Autodesk Fusion 360 part; units mm, degrees
note: some values were not read from the file. Set by a fixed rule: which sketch regions a step uses.
(part 3 of 4)
sketch "スケッチ30" plane through (0, 0, 3) normal (0, 0, 1) x (-1, 0, 0)
  arc A0 (40, -80.2208) -> (44, -84.2208) centre (44, -80.2208) ccw
  line L0 (44, -84.2208) -> (61.0153, -84.2208)
  arc A1 (61.0153, -84.2208) -> (67.021, -79.5248) centre (0, 0) ccw
  arc A2 (67.021, -79.5248) -> (66.4432, -73.002) centre (64.4432, -76.4661) ccw
  line L1 (66.4432, -73.002) -> (56.3605, -67.1808)
  arc A3 (55.6284, -64.4487) -> (56.3605, -67.1808) centre (57.3605, -65.4487) ccw
  line L2 (55.6284, -64.4487) -> (83.6284, -15.9513)
  arc A4 (86.3605, -15.2192) -> (83.6284, -15.9513) centre (85.3605, -16.9513) ccw
  line L3 (86.3605, -15.2192) -> (96.4432, -21.0405)
  arc A5 (96.4432, -21.0405) -> (102.381, -18.2795) centre (98.4432, -17.5764) ccw
  arc A6 (102.381, -18.2795) -> (94.1613, 44.1547) centre (0, 0) ccw
  arc A7 (94.1613, 44.1547) -> (87.7113, 45.2849) centre (90.5398, 42.4565) ccw
  line L4 (87.7113, 45.2849) -> (79.4788, 37.0524)
  arc A8 (76.6504, 37.0524) -> (79.4788, 37.0524) centre (78.0646, 38.4666) ccw
  line L5 (76.6504, 37.0524) -> (37.0524, 76.6504)
  arc A9 (37.0524, 79.4788) -> (37.0524, 76.6504) centre (38.4666, 78.0646) ccw
  line L6 (37.0524, 79.4788) -> (45.2849, 87.7113)
  arc A10 (45.2849, 87.7113) -> (44.1547, 94.1613) centre (42.4565, 90.5398) ccw
  arc A11 (44.1547, 94.1613) -> (-44.1547, 94.1613) centre (0, 0) ccw
  arc A12 (-44.1547, 94.1613) -> (-45.2849, 87.7113) centre (-42.4565, 90.5398) ccw
  line L7 (-45.2849, 87.7113) -> (-37.0524, 79.4788)
  arc A13 (-37.0524, 76.6504) -> (-37.0524, 79.4788) centre (-38.4666, 78.0646) ccw
  line L8 (-37.0524, 76.6504) -> (-76.6504, 37.0524)
  arc A14 (-79.4788, 37.0524) -> (-76.6504, 37.0524) centre (-78.0646, 38.4666) ccw
  line L9 (-79.4788, 37.0524) -> (-87.7113, 45.2849)
  arc A15 (-87.7113, 45.2849) -> (-94.1613, 44.1547) centre (-90.5398, 42.4565) ccw
  arc A16 (-94.1613, 44.1547) -> (-102.381, -18.2795) centre (0, 0) ccw
  arc A17 (-102.381, -18.2795) -> (-96.4432, -21.0405) centre (-98.4432, -17.5764) ccw
  line L10 (-96.4432, -21.0405) -> (-86.3605, -15.2192)
  arc A18 (-83.6284, -15.9513) -> (-86.3605, -15.2192) centre (-85.3605, -16.9513) ccw
  line L11 (-83.6284, -15.9513) -> (-55.6284, -64.4487)
  arc A19 (-56.3605, -67.1808) -> (-55.6284, -64.4487) centre (-57.3605, -65.4487) ccw
  line L12 (-56.3605, -67.1808) -> (-66.4432, -73.002)
  arc A20 (-66.4432, -73.002) -> (-67.021, -79.5248) centre (-64.4432, -76.4661) ccw
  arc A21 (-67.021, -79.5248) -> (-61.3188, -84) centre (0, 0) ccw
  line L13 (-61.3188, -84) -> (-44, -84)
  arc A22 (-44, -84) -> (-40, -80) centre (-44, -80) ccw
  line L14 (-40, -80) -> (-40, -66)
  arc A23 (-38, -64) -> (-40, -66) centre (-38, -66) ccw
  line L15 (-38, -64) -> (38, -64)
  arc A24 (40, -66) -> (38, -64) centre (38, -66) ccw
  line L16 (40, -66) -> (40, -80.2208)
  arc A25 (-4, -46.6154) -> (-5.7447, -44.6318) centre (-6, -46.6154) ccw
  arc A26 (-28.3589, -34.9396) -> (-5.7447, -44.6318) centre (0, 0) ccw
  arc A27 (-28.4908, -31.9509) -> (-28.3589, -34.9396) centre (-27.0985, -33.3867) ccw
  line L17 (-28.4908, -31.9509) -> (-25.5966, -29.1445)
  arc A28 (-22.9631, -29.012) -> (-25.5966, -29.1445) centre (-24.2043, -30.5803) ccw
  arc A29 (-22.9631, -29.012) -> (22.9694, -29.007) centre (0, 0) ccw
  arc A30 (25.6252, -29.1607) -> (22.9694, -29.007) centre (24.211, -30.575) ccw
  line L18 (25.6252, -29.1607) -> (28.4709, -32.0064)
  arc A31 (28.3151, -34.9751) -> (28.4709, -32.0064) centre (27.0567, -33.4206) ccw
  arc A32 (5.7447, -44.6318) -> (28.3151, -34.9751) centre (0, 0) ccw
  arc A33 (5.7447, -44.6318) -> (4, -46.6154) centre (6, -46.6154) ccw
  line L19 (4, -46.6154) -> (4, -48)
  arc A34 (4, -48) -> (6, -50) centre (6, -48) ccw
  line L20 (6, -50) -> (38, -50)
  arc A35 (40, -52) -> (38, -50) centre (38, -52) ccw
  line L21 (40, -52) -> (40, -56)
  arc A36 (38, -58) -> (40, -56) centre (38, -56) ccw
  line L22 (38, -58) -> (-38, -58)
  arc A37 (-40, -56) -> (-38, -58) centre (-38, -56) ccw
  line L23 (-40, -56) -> (-40, -52)
  arc A38 (-38, -50) -> (-40, -52) centre (-38, -52) ccw
  line L24 (-38, -50) -> (-6, -50)
  arc A39 (-6, -50) -> (-4, -48) centre (-6, -48) ccw
  line L25 (-4, -48) -> (-4, -47)
  line L26 (-4, -47) -> (-4, -46.6154)
  line L27 (55.9233, -53.938) -> (50.6914, -63)
  arc A40 (48.9593, -64) -> (50.6914, -63) centre (48.9593, -62) ccw
  line L28 (48.9593, -64) -> (47, -64)
  arc A41 (45, -62) -> (47, -64) centre (47, -62) ccw
  line L29 (45, -62) -> (45, -51.9629)
  arc A42 (46.9625, -49.9632) -> (45, -51.9629) centre (47, -51.9629) ccw
  line L30 (46.9625, -49.9632) -> (52.2919, -49.8634)
  arc A43 (53.3294, -50.131) -> (52.2919, -49.8634) centre (52.3294, -51.863) ccw
  line L31 (53.3294, -50.131) -> (55.1913, -51.2059)
  arc A44 (55.9233, -53.938) -> (55.1913, -51.2059) centre (54.1913, -52.938) ccw
  line L32 (-52.5666, -50) -> (-47, -50)
  arc A45 (-45, -52) -> (-47, -50) centre (-47, -52) ccw
  line L33 (-45, -52) -> (-45, -62)
  arc A46 (-47, -64) -> (-45, -62) centre (-47, -62) ccw
  line L34 (-47, -64) -> (-48.9593, -64)
  arc A47 (-50.6914, -63) -> (-48.9593, -64) centre (-48.9593, -62) ccw
  line L35 (-50.6914, -63) -> (-55.9233, -53.938)
  arc A48 (-55.1913, -51.2059) -> (-55.9233, -53.938) centre (-54.1913, -52.938) ccw
  line L36 (-55.1913, -51.2059) -> (-53.5666, -50.2679)
  arc A49 (-52.5666, -50) -> (-53.5666, -50.2679) centre (-52.5666, -52) ccw
  arc A50 (76.6504, 29.9813) -> (79.4788, 29.9813) centre (78.0646, 31.3955) ccw
  line L37 (79.4788, 29.9813) -> (88.1522, 38.6547)
  arc A51 (91.4132, 38.0084) -> (88.1522, 38.6547) centre (89.5664, 37.2405) ccw
  arc A52 (98.3614, 11.2268) -> (91.4132, 38.0084) centre (0, 0) ccw
  arc A53 (96.3743, 9) -> (98.3614, 11.2268) centre (96.3743, 11) ccw
  line L38 (96.3743, 9) -> (50.8232, 9)
  arc A54 (48.8685, 10.5769) -> (50.8232, 9) centre (50.8232, 11) ccw
  arc A55 (48.8685, 10.5769) -> (45.7253, 20.2286) centre (0, 0) ccw
  arc A56 (46.1401, 22.452) -> (45.7253, 20.2286) centre (47.5543, 21.0378) ccw
  line L39 (46.1401, 22.452) -> (63.7457, 40.0576)
  arc A57 (66.5741, 40.0576) -> (63.7457, 40.0576) centre (65.1599, 38.6434) ccw
  line L40 (66.5741, 40.0576) -> (76.6504, 29.9813)
  arc A58 (98.1356, -13.0538) -> (98.3593, -11.2453) centre (0, 0) ccw
  arc A59 (95.1531, -14.5221) -> (98.1356, -13.0538) centre (96.1531, -12.7901) ccw
  line L41 (95.1531, -14.5221) -> (92.084, -12.7502)
  arc A60 (93.084, -9.0182) -> (92.084, -12.7502) centre (93.084, -11.0182) ccw
  line L42 (93.084, -9.0182) -> (96.3722, -9.0182)
  arc A61 (98.3593, -11.2453) -> (96.3722, -9.0182) centre (96.3722, -11.0182) ccw
  line L43 (-96.3722, -9.0182) -> (-93.084, -9.0182)
  arc A62 (-92.084, -12.7502) -> (-93.084, -9.0182) centre (-93.084, -11.0182) ccw
  line L44 (-92.084, -12.7502) -> (-95.1531, -14.5221)
  arc A63 (-98.1356, -13.0538) -> (-95.1531, -14.5221) centre (-96.1531, -12.7901) ccw
  arc A64 (-98.3593, -11.2453) -> (-98.1356, -13.0538) centre (0, 0) ccw
  arc A65 (-96.3722, -9.0182) -> (-98.3593, -11.2453) centre (-96.3722, -11.0182) ccw
  arc A66 (-44.6318, -5.7447) -> (-46.6154, -4) centre (-46.6154, -6) ccw
  line L45 (-46.6154, -4) -> (-96.9794, -4)
  arc A67 (-98.979, -2.0412) -> (-96.9794, -4) centre (-96.9794, -2) ccw
  arc A68 (-98.979, 2.0412) -> (-98.979, -2.0412) centre (0, 0) ccw
  arc A69 (-96.9794, 4) -> (-98.979, 2.0412) centre (-96.9794, 2) ccw
  line L46 (-96.9794, 4) -> (-46.6154, 4)
  arc A70 (-46.6154, 4) -> (-44.6318, 5.7447) centre (-46.6154, 6) ccw
  arc A71 (-34.9648, 28.3278) -> (-44.6318, 5.7447) centre (0, 0) ccw
  arc A72 (-31.975, 28.4611) -> (-34.9648, 28.3278) centre (-33.4108, 27.0688) ccw
  line L47 (-31.975, 28.4611) -> (-29.1682, 25.5666)
  arc A73 (-29.0345, 22.9346) -> (-29.1682, 25.5666) centre (-30.604, 24.1743) ccw
  arc A74 (-29.0345, 22.9346) -> (-29.007, -22.9694) centre (0, 0) ccw
  arc A75 (-29.1607, -25.6252) -> (-29.007, -22.9694) centre (-30.575, -24.211) ccw
  line L48 (-29.1607, -25.6252) -> (-32.0064, -28.4709)
  arc A76 (-34.9751, -28.3151) -> (-32.0064, -28.4709) centre (-33.4206, -27.0567) ccw
  arc A77 (-44.6318, -5.7447) -> (-34.9751, -28.3151) centre (0, 0) ccw
  line L49 (27.8089, 44.4259) -> (43.5931, 60.2101)
  arc A78 (46.4216, 60.2101) -> (43.5931, 60.2101) centre (45.0073, 58.7959) ccw
  line L50 (46.4216, 60.2101) -> (60.2101, 46.4216)
  arc A79 (60.2101, 43.5931) -> (60.2101, 46.4216) centre (58.7959, 45.0073) ccw
  line L51 (60.2101, 43.5931) -> (44.4259, 27.8089)
  arc A80 (41.3574, 28.0992) -> (44.4259, 27.8089) centre (43.0117, 29.2231) ccw
  arc A81 (41.3574, 28.0992) -> (28.0992, 41.3574) centre (0, 0) ccw
  arc A82 (27.8089, 44.4259) -> (28.0992, 41.3574) centre (29.2231, 43.0117) ccw
  line L52 (-38.3596, -35.7147) -> (-57.6913, -46.8758)
  arc A83 (-60.4233, -46.1437) -> (-57.6913, -46.8758) centre (-58.6913, -45.1437) ccw
  line L53 (-60.4233, -46.1437) -> (-70.1733, -29.2563)
  arc A84 (-69.4413, -26.5242) -> (-70.1733, -29.2563) centre (-68.4413, -28.2563) ccw
  line L54 (-69.4413, -26.5242) -> (-50.1096, -15.3631)
  arc A85 (-47.2208, -16.4376) -> (-50.1096, -15.3631) centre (-49.1096, -17.0951) ccw
  arc A86 (-47.2208, -16.4376) -> (-37.8458, -32.6756) centre (0, 0) ccw
  arc A87 (-38.3596, -35.7147) -> (-37.8458, -32.6756) centre (-39.3596, -33.9826) ccw
  arc A88 (-31.3739, -38.9317) -> (-28.1158, -41.3462) centre (0, 0) ccw
  arc A89 (-29.2404, -45) -> (-28.1158, -41.3462) centre (-29.2404, -43) ccw
  line L55 (-29.2404, -45) -> (-36.9782, -45)
  arc A90 (-37.9782, -41.2679) -> (-36.9782, -45) centre (-36.9782, -43) ccw
  line L56 (-37.9782, -41.2679) -> (-33.6289, -38.7569)
  arc A91 (-31.3739, -38.9317) -> (-33.6289, -38.7569) centre (-32.6289, -40.4889) ccw
  line L57 (80.1362, -12) -> (74.6733, -21.462)
  arc A92 (71.9413, -22.1941) -> (74.6733, -21.462) centre (72.9413, -20.462) ccw
  line L58 (71.9413, -22.1941) -> (55.6136, -12.7673)
  arc A93 (56.6098, -9.0353) -> (55.6136, -12.7673) centre (56.6136, -11.0353) ccw
  line L59 (56.6098, -9.0353) -> (75, -9)
  line L60 (75, -9) -> (78.4042, -9)
  arc A94 (80.1362, -12) -> (78.4042, -9) centre (78.4042, -11) ccw
  line L61 (-44.4259, 27.8089) -> (-60.2101, 43.5931)
  arc A95 (-60.2101, 46.4216) -> (-60.2101, 43.5931) centre (-58.7959, 45.0073) ccw
  line L62 (-60.2101, 46.4216) -> (-46.4216, 60.2101)
  arc A96 (-43.5931, 60.2101) -> (-46.4216, 60.2101) centre (-45.0073, 58.7959) ccw
  line L63 (-43.5931, 60.2101) -> (-27.8089, 44.4259)
  arc A97 (-28.0992, 41.3574) -> (-27.8089, 44.4259) centre (-29.2231, 43.0117) ccw
  arc A98 (-28.0992, 41.3574) -> (-41.3574, 28.0992) centre (0, 0) ccw
  arc A99 (-44.4259, 27.8089) -> (-41.3574, 28.0992) centre (-43.0117, 29.2231) ccw
  line L64 (50.1096, -15.3631) -> (69.4413, -26.5242)
  arc A100 (70.1733, -29.2563) -> (69.4413, -26.5242) centre (68.4413, -28.2563) ccw
  line L65 (70.1733, -29.2563) -> (60.4233, -46.1437)
  arc A101 (57.6913, -46.8758) -> (60.4233, -46.1437) centre (58.6913, -45.1437) ccw
  line L66 (57.6913, -46.8758) -> (38.3596, -35.7147)
  arc A102 (37.8458, -32.6756) -> (38.3596, -35.7147) centre (39.3596, -33.9826) ccw
  arc A103 (37.8458, -32.6756) -> (47.2208, -16.4376) centre (0, 0) ccw
  arc A104 (50.1096, -15.3631) -> (47.2208, -16.4376) centre (49.1096, -17.0951) ccw
  line L67 (-78.4041, -8.9935) -> (-56.6098, -9.0353)
  arc A105 (-55.6136, -12.7673) -> (-56.6098, -9.0353) centre (-56.6136, -11.0353) ccw
  line L68 (-55.6136, -12.7673) -> (-71.9413, -22.1941)
  arc A106 (-74.6733, -21.462) -> (-71.9413, -22.1941) centre (-72.9413, -20.462) ccw
  line L69 (-74.6733, -21.462) -> (-80.14, -11.9935)
  arc A107 (-78.4041, -8.9935) -> (-80.14, -11.9935) centre (-78.4079, -10.9935) ccw
  line L70 (33.6289, -38.7569) -> (37.9782, -41.268)
  arc A108 (36.9782, -45) -> (37.9782, -41.268) centre (36.9782, -43) ccw
  line L71 (36.9782, -45) -> (29.2404, -45)
  arc A109 (28.1158, -41.3462) -> (29.2404, -45) centre (29.2404, -43) ccw
  arc A110 (28.1158, -41.3462) -> (31.3739, -38.9317) centre (0, 0) ccw
  arc A111 (33.6289, -38.7569) -> (31.3739, -38.9317) centre (32.6289, -40.4889) ccw
  circle A112 centre (0, 0) radius 32
  circle A113 centre (-51.2451, -46.0409) radius 1.5
  circle A114 centre (51.2451, -46.0409) radius 1.5
  circle A115 centre (-65.4951, -21.3591) radius 1.5
  circle A116 centre (-57.7353, 37.5827) radius 1.5
  circle A117 centre (-37.5827, 57.7353) radius 1.5
  circle A118 centre (37.5827, 57.7353) radius 1.5
  circle A119 centre (57.7353, 37.5827) radius 1.5
  circle A120 centre (65.4951, -21.3591) radius 1.5
  arc A121 (46.6154, -4) -> (44.6318, -5.7447) centre (46.6154, -6) ccw
  arc A122 (34.9751, -28.3151) -> (44.6318, -5.7447) centre (0, 0) ccw
  arc A123 (32.0064, -28.4709) -> (34.9751, -28.3151) centre (33.4206, -27.0567) ccw
  line L72 (32.0064, -28.4709) -> (29.1607, -25.6252)
  arc A124 (29.007, -22.9694) -> (29.1607, -25.6252) centre (30.575, -24.211) ccw
  arc A125 (29.007, -22.9694) -> (29.007, 22.9694) centre (0, 0) ccw
  arc A126 (29.1607, 25.6252) -> (29.007, 22.9694) centre (30.575, 24.211) ccw
  line L73 (29.1607, 25.6252) -> (32.0064, 28.4709)
  arc A127 (34.9751, 28.3151) -> (32.0064, 28.4709) centre (33.4206, 27.0567) ccw
  arc A128 (44.6318, 5.7447) -> (34.9751, 28.3151) centre (0, 0) ccw
  arc A129 (44.6318, 5.7447) -> (46.6154, 4) centre (46.6154, 6) ccw
  line L74 (46.6154, 4) -> (96.9794, 4)
  arc A130 (98.979, 2.0412) -> (96.9794, 4) centre (96.9794, 2) ccw
  arc A131 (98.979, -2.0412) -> (98.979, 2.0412) centre (0, 0) ccw
  arc A132 (96.9794, -4) -> (98.979, -2.0412) centre (96.9794, -2) ccw
  line L75 (96.9794, -4) -> (46.6154, -4)
  arc A133 (-5.7447, 44.6318) -> (-4, 46.6154) centre (-6, 46.6154) ccw
  line L76 (-4, 46.6154) -> (-4, 96.9794)
  arc A134 (-2.0412, 98.979) -> (-4, 96.9794) centre (-2, 96.9794) ccw
  arc A135 (2.0412, 98.979) -> (-2.0412, 98.979) centre (0, 0) ccw
  arc A136 (4, 96.9794) -> (2.0412, 98.979) centre (2, 96.9794) ccw
  line L77 (4, 96.9794) -> (4, 46.6154)
  arc A137 (4, 46.6154) -> (5.7447, 44.6318) centre (6, 46.6154) ccw
  arc A138 (28.3151, 34.9751) -> (5.7447, 44.6318) centre (0, 0) ccw
  arc A139 (28.4709, 32.0064) -> (28.3151, 34.9751) centre (27.0567, 33.4206) ccw
  line L78 (28.4709, 32.0064) -> (25.6252, 29.1607)
  arc A140 (22.9694, 29.007) -> (25.6252, 29.1607) centre (24.211, 30.575) ccw
  arc A141 (22.9694, 29.007) -> (-22.9694, 29.007) centre (0, 0) ccw
  arc A142 (-25.6252, 29.1607) -> (-22.9694, 29.007) centre (-24.211, 30.575) ccw
  line L79 (-25.6252, 29.1607) -> (-28.4709, 32.0064)
  arc A143 (-28.3151, 34.9751) -> (-28.4709, 32.0064) centre (-27.0567, 33.4206) ccw
  arc A144 (-5.7447, 44.6318) -> (-28.3151, 34.9751) centre (0, 0) ccw
  arc A145 (31.3955, 80.893) -> (31.3955, 75.2362) centre (34.224, 78.0646) ccw
  line L80 (31.3955, 75.2362) -> (40.0576, 66.5741)
  arc A146 (40.0576, 63.7457) -> (40.0576, 66.5741) centre (38.6434, 65.1599) ccw
  line L81 (40.0576, 63.7457) -> (22.452, 46.1401)
  arc A147 (20.2286, 45.7253) -> (22.452, 46.1401) centre (21.0378, 47.5543) ccw
  arc A148 (20.2286, 45.7253) -> (10.5769, 48.8685) centre (0, 0) ccw
  arc A149 (9, 50.8232) -> (10.5769, 48.8685) centre (11, 50.8232) ccw
  line L82 (9, 50.8232) -> (9, 96.3743)
  arc A150 (11.2268, 98.3614) -> (9, 96.3743) centre (11, 96.3743) ccw
  arc A151 (38.0084, 91.4132) -> (11.2268, 98.3614) centre (0, 0) ccw
  arc A152 (38.6547, 88.1522) -> (38.0084, 91.4132) centre (37.2405, 89.5664) ccw
  line L83 (38.6547, 88.1522) -> (31.3955, 80.893)
  arc A153 (-31.3955, 75.2362) -> (-31.3955, 80.893) centre (-34.224, 78.0646) ccw
  line L84 (-31.3955, 80.893) -> (-38.6547, 88.1522)
  arc A154 (-38.0084, 91.4132) -> (-38.6547, 88.1522) centre (-37.2405, 89.5664) ccw
  arc A155 (-11.2268, 98.3614) -> (-38.0084, 91.4132) centre (0, 0) ccw
  arc A156 (-9, 96.3743) -> (-11.2268, 98.3614) centre (-11, 96.3743) ccw
  line L85 (-9, 96.3743) -> (-9, 50.8232)
  arc A157 (-10.5769, 48.8685) -> (-9, 50.8232) centre (-11, 50.8232) ccw
  arc A158 (-10.5769, 48.8685) -> (-20.2286, 45.7253) centre (0, 0) ccw
  arc A159 (-22.452, 46.1401) -> (-20.2286, 45.7253) centre (-21.0378, 47.5543) ccw
  line L86 (-22.452, 46.1401) -> (-40.0576, 63.7457)
  arc A160 (-40.0576, 66.5741) -> (-40.0576, 63.7457) centre (-38.6434, 65.1599) ccw
  line L87 (-40.0576, 66.5741) -> (-31.3955, 75.2362)
  arc A161 (-80.893, 31.3955) -> (-75.2362, 31.3955) centre (-78.0646, 34.224) ccw
  line L88 (-75.2362, 31.3955) -> (-66.5741, 40.0576)
  arc A162 (-63.7457, 40.0576) -> (-66.5741, 40.0576) centre (-65.1599, 38.6434) ccw
  line L89 (-63.7457, 40.0576) -> (-46.1401, 22.452)
  arc A163 (-45.7253, 20.2286) -> (-46.1401, 22.452) centre (-47.5543, 21.0378) ccw
  arc A164 (-45.7253, 20.2286) -> (-48.8685, 10.5769) centre (0, 0) ccw
  arc A165 (-50.8232, 9) -> (-48.8685, 10.5769) centre (-50.8232, 11) ccw
  line L90 (-50.8232, 9) -> (-96.3743, 9)
  arc A166 (-98.3614, 11.2268) -> (-96.3743, 9) centre (-96.3743, 11) ccw
  arc A167 (-91.4132, 38.0084) -> (-98.3614, 11.2268) centre (0, 0) ccw
  arc A168 (-88.1522, 38.6547) -> (-91.4132, 38.0084) centre (-89.5664, 37.2405) ccw
  line L91 (-88.1522, 38.6547) -> (-80.893, 31.3955)
  line L92 (0, -64) -> (0, -84)
  line L93 (0, -84) -> (68, -84)
  line L94 (61.3188, -84) -> (60.734, -84.4269)
  line L95 (61.0153, -84.2208) -> (39.7351, -84.2208)
  line L96 (39.7351, -84.2208) -> (39.5, -84)
  constraint midpoint L15 L92.start
  constraint perpendicular L15 L92
  constraint perpendicular L92 L93
  constraint coincident A1 L94.start
  constraint coincident L93 L94.start
  constraint tangent A1 L94
  constraint coincident L0.end A1.start
  constraint parallel L0 L95
  constraint coincident L93 L96.end
delete_face "面を削除4" 1 faces at (-40.4447, 82.0537, 2.5) on bodies 1
extrude "押し出し29" cut sketch "スケッチ30" against normal blind 6 contours A0 L0 A1 L93 L94 L95 | A0 L93 L95 L96 bodies 1
fillet "フィレット31" radius 4 1 edges at (-40, 84, 2.25) on bodies 1
fillet "フィレット32" radius 19.01 1 edges at (61.3188, 84, 2.25) on bodies 1
fillet "フィレット33" radius 19.01 1 edges at (-61.3188, 84, 2.25) on bodies 1
sketch "スケッチ31" plane through (0, 0, 3) normal (0, 0, 1) x (-1, 0, 0)
  arc A0 (54.7686, -84) -> (67.0189, -79.5265) centre (54.7686, -64.99) ccw
  arc A1 (67.0189, -79.5265) -> (67.021, -79.5248) centre (0, 0) ccw
  arc A2 (67.021, -79.5248) -> (66.4432, -73.002) centre (64.4432, -76.4661) ccw
  line L0 (66.4432, -73.002) -> (56.3605, -67.1808)
  arc A3 (55.6284, -64.4487) -> (56.3605, -67.1808) centre (57.3605, -65.4487) ccw
  line L1 (55.6284, -64.4487) -> (83.6284, -15.9513)
  arc A4 (86.3605, -15.2192) -> (83.6284, -15.9513) centre (85.3605, -16.9513) ccw
  line L2 (86.3605, -15.2192) -> (96.4432, -21.0405)
  arc A5 (96.4432, -21.0405) -> (102.381, -18.2795) centre (98.4432, -17.5764) ccw
  arc A6 (102.381, -18.2795) -> (94.1613, 44.1547) centre (0, 0) ccw
  arc A7 (94.1613, 44.1547) -> (87.7113, 45.2849) centre (90.5398, 42.4565) ccw
  line L3 (87.7113, 45.2849) -> (79.4788, 37.0524)
  arc A8 (76.6504, 37.0524) -> (79.4788, 37.0524) centre (78.0646, 38.4666) ccw
  line L4 (76.6504, 37.0524) -> (37.0524, 76.6504)
  arc A9 (37.0524, 79.4788) -> (37.0524, 76.6504) centre (38.4666, 78.0646) ccw
  line L5 (37.0524, 79.4788) -> (45.2849, 87.7113)
  arc A10 (45.2849, 87.7113) -> (44.1547, 94.1613) centre (42.4565, 90.5398) ccw
  arc A11 (44.1547, 94.1613) -> (-44.1547, 94.1613) centre (0, 0) ccw
  arc A12 (-44.1547, 94.1613) -> (-45.2849, 87.7113) centre (-42.4565, 90.5398) ccw
  line L6 (-45.2849, 87.7113) -> (-37.0524, 79.4788)
  arc A13 (-37.0524, 76.6504) -> (-37.0524, 79.4788) centre (-38.4666, 78.0646) ccw
  line L7 (-37.0524, 76.6504) -> (-76.6504, 37.0524)
  arc A14 (-79.4788, 37.0524) -> (-76.6504, 37.0524) centre (-78.0646, 38.4666) ccw
  line L8 (-79.4788, 37.0524) -> (-87.7113, 45.2849)
  arc A15 (-87.7113, 45.2849) -> (-94.1613, 44.1547) centre (-90.5398, 42.4565) ccw
  arc A16 (-94.1613, 44.1547) -> (-102.381, -18.2795) centre (0, 0) ccw
  arc A17 (-102.381, -18.2795) -> (-96.4432, -21.0405) centre (-98.4432, -17.5764) ccw
  line L9 (-96.4432, -21.0405) -> (-86.3605, -15.2192)
  arc A18 (-83.6284, -15.9513) -> (-86.3605, -15.2192) centre (-85.3605, -16.9513) ccw
  line L10 (-83.6284, -15.9513) -> (-55.6284, -64.4487)
  arc A19 (-56.3605, -67.1808) -> (-55.6284, -64.4487) centre (-57.3605, -65.4487) ccw
  line L11 (-56.3605, -67.1808) -> (-66.4432, -73.002)
  arc A20 (-66.4432, -73.002) -> (-67.021, -79.5248) centre (-64.4432, -76.4661) ccw
  arc A21 (-67.021, -79.5248) -> (-67.0189, -79.5265) centre (0.0001, 0.0001) ccw
  arc A22 (-67.0189, -79.5265) -> (-54.7686, -84) centre (-54.7686, -64.99) ccw
  line L12 (-54.7686, -84) -> (-44, -84)
  arc A23 (-44, -84) -> (-40, -80) centre (-44, -80) ccw
  line L13 (-40, -80) -> (-40, -66)
  arc A24 (-38, -64) -> (-40, -66) centre (-38, -66) ccw
  line L14 (-38, -64) -> (38, -64)
  arc A25 (40, -66) -> (38, -64) centre (38, -66) ccw
  line L15 (40, -66) -> (40, -80)
  arc A26 (40, -80) -> (44, -84) centre (44, -80) ccw
  line L16 (44, -84) -> (54.7686, -84)
  arc A27 (-4, -46.6154) -> (-5.7447, -44.6318) centre (-6, -46.6154) ccw
  arc A28 (-28.3589, -34.9396) -> (-5.7447, -44.6318) centre (0, 0) ccw
  arc A29 (-28.4908, -31.9509) -> (-28.3589, -34.9396) centre (-27.0985, -33.3867) ccw
  line L17 (-28.4908, -31.9509) -> (-25.5966, -29.1445)
  arc A30 (-22.9631, -29.012) -> (-25.5966, -29.1445) centre (-24.2043, -30.5803) ccw
  arc A31 (-22.9631, -29.012) -> (22.9694, -29.007) centre (0, 0) ccw
  arc A32 (25.6252, -29.1607) -> (22.9694, -29.007) centre (24.211, -30.575) ccw
  line L18 (25.6252, -29.1607) -> (28.4709, -32.0064)
  arc A33 (28.3151, -34.9751) -> (28.4709, -32.0064) centre (27.0567, -33.4206) ccw
  arc A34 (5.7447, -44.6318) -> (28.3151, -34.9751) centre (0, 0) ccw
  arc A35 (5.7447, -44.6318) -> (4, -46.6154) centre (6, -46.6154) ccw
  line L19 (4, -46.6154) -> (4, -48)
  arc A36 (4, -48) -> (6, -50) centre (6, -48) ccw
  line L20 (6, -50) -> (38, -50)
  arc A37 (40, -52) -> (38, -50) centre (38, -52) ccw
  line L21 (40, -52) -> (40, -56)
  arc A38 (38, -58) -> (40, -56) centre (38, -56) ccw
  line L22 (38, -58) -> (-38, -58)
  arc A39 (-40, -56) -> (-38, -58) centre (-38, -56) ccw
  line L23 (-40, -56) -> (-40, -52)
  arc A40 (-38, -50) -> (-40, -52) centre (-38, -52) ccw
  line L24 (-38, -50) -> (-6, -50)
  arc A41 (-6, -50) -> (-4, -48) centre (-6, -48) ccw
  line L25 (-4, -48) -> (-4, -47)
  line L26 (-4, -47) -> (-4, -46.6154)
  line L27 (55.9233, -53.938) -> (50.6914, -63)
  arc A42 (48.9593, -64) -> (50.6914, -63) centre (48.9593, -62) ccw
  line L28 (48.9593, -64) -> (47, -64)
  arc A43 (45, -62) -> (47, -64) centre (47, -62) ccw
  line L29 (45, -62) -> (45, -51.9629)
  arc A44 (46.9625, -49.9632) -> (45, -51.9629) centre (47, -51.9629) ccw
  line L30 (46.9625, -49.9632) -> (52.2919, -49.8634)
  arc A45 (53.3294, -50.131) -> (52.2919, -49.8634) centre (52.3294, -51.863) ccw
  line L31 (53.3294, -50.131) -> (55.1913, -51.2059)
  arc A46 (55.9233, -53.938) -> (55.1913, -51.2059) centre (54.1913, -52.938) ccw
  line L32 (-52.5666, -50) -> (-47, -50)
  arc A47 (-45, -52) -> (-47, -50) centre (-47, -52) ccw
  line L33 (-45, -52) -> (-45, -62)
  arc A48 (-47, -64) -> (-45, -62) centre (-47, -62) ccw
  line L34 (-47, -64) -> (-48.9593, -64)
  arc A49 (-50.6914, -63) -> (-48.9593, -64) centre (-48.9593, -62) ccw
  line L35 (-50.6914, -63) -> (-55.9233, -53.938)
  arc A50 (-55.1913, -51.2059) -> (-55.9233, -53.938) centre (-54.1913, -52.938) ccw
  line L36 (-55.1913, -51.2059) -> (-53.5666, -50.2679)
  arc A51 (-52.5666, -50) -> (-53.5666, -50.2679) centre (-52.5666, -52) ccw
  arc A52 (76.6504, 29.9813) -> (79.4788, 29.9813) centre (78.0646, 31.3955) ccw
  line L37 (79.4788, 29.9813) -> (88.1522, 38.6547)
  arc A53 (91.4132, 38.0084) -> (88.1522, 38.6547) centre (89.5664, 37.2405) ccw
  arc A54 (98.3614, 11.2268) -> (91.4132, 38.0084) centre (0, 0) ccw
  arc A55 (96.3743, 9) -> (98.3614, 11.2268) centre (96.3743, 11) ccw
  line L38 (96.3743, 9) -> (50.8232, 9)
  arc A56 (48.8685, 10.5769) -> (50.8232, 9) centre (50.8232, 11) ccw
  arc A57 (48.8685, 10.5769) -> (45.7253, 20.2286) centre (0, 0) ccw
  arc A58 (46.1401, 22.452) -> (45.7253, 20.2286) centre (47.5543, 21.0378) ccw
  line L39 (46.1401, 22.452) -> (63.7457, 40.0576)
  arc A59 (66.5741, 40.0576) -> (63.7457, 40.0576) centre (65.1599, 38.6434) ccw
  line L40 (66.5741, 40.0576) -> (76.6504, 29.9813)
  arc A60 (98.1356, -13.0538) -> (98.3593, -11.2453) centre (0, 0) ccw
  arc A61 (95.1531, -14.5221) -> (98.1356, -13.0538) centre (96.1531, -12.7901) ccw
  line L41 (95.1531, -14.5221) -> (92.084, -12.7502)
  arc A62 (93.084, -9.0182) -> (92.084, -12.7502) centre (93.084, -11.0182) ccw
  line L42 (93.084, -9.0182) -> (96.3722, -9.0182)
  arc A63 (98.3593, -11.2453) -> (96.3722, -9.0182) centre (96.3722, -11.0182) ccw
  line L43 (-96.3722, -9.0182) -> (-93.084, -9.0182)
  arc A64 (-92.084, -12.7502) -> (-93.084, -9.0182) centre (-93.084, -11.0182) ccw
  line L44 (-92.084, -12.7502) -> (-95.1531, -14.5221)
  arc A65 (-98.1356, -13.0538) -> (-95.1531, -14.5221) centre (-96.1531, -12.7901) ccw
  arc A66 (-98.3593, -11.2453) -> (-98.1356, -13.0538) centre (0, 0) ccw
  arc A67 (-96.3722, -9.0182) -> (-98.3593, -11.2453) centre (-96.3722, -11.0182) ccw
  arc A68 (-44.6318, -5.7447) -> (-46.6154, -4) centre (-46.6154, -6) ccw
  line L45 (-46.6154, -4) -> (-96.9794, -4)
  arc A69 (-98.979, -2.0412) -> (-96.9794, -4) centre (-96.9794, -2) ccw
  arc A70 (-98.979, 2.0412) -> (-98.979, -2.0412) centre (0, 0) ccw
  arc A71 (-96.9794, 4) -> (-98.979, 2.0412) centre (-96.9794, 2) ccw
  line L46 (-96.9794, 4) -> (-46.6154, 4)
  arc A72 (-46.6154, 4) -> (-44.6318, 5.7447) centre (-46.6154, 6) ccw
  arc A73 (-34.9648, 28.3278) -> (-44.6318, 5.7447) centre (0, 0) ccw
  arc A74 (-31.975, 28.4611) -> (-34.9648, 28.3278) centre (-33.4108, 27.0688) ccw
  line L47 (-31.975, 28.4611) -> (-29.1682, 25.5666)
  arc A75 (-29.0345, 22.9346) -> (-29.1682, 25.5666) centre (-30.604, 24.1743) ccw
  arc A76 (-29.0345, 22.9346) -> (-29.007, -22.9694) centre (0, 0) ccw
  arc A77 (-29.1607, -25.6252) -> (-29.007, -22.9694) centre (-30.575, -24.211) ccw
  line L48 (-29.1607, -25.6252) -> (-32.0064, -28.4709)
  arc A78 (-34.9751, -28.3151) -> (-32.0064, -28.4709) centre (-33.4206, -27.0567) ccw
  arc A79 (-44.6318, -5.7447) -> (-34.9751, -28.3151) centre (0, 0) ccw
  line L49 (27.8089, 44.4259) -> (43.5931, 60.2101)
  arc A80 (46.4216, 60.2101) -> (43.5931, 60.2101) centre (45.0073, 58.7959) ccw
  line L50 (46.4216, 60.2101) -> (60.2101, 46.4216)
  arc A81 (60.2101, 43.5931) -> (60.2101, 46.4216) centre (58.7959, 45.0073) ccw
  line L51 (60.2101, 43.5931) -> (44.4259, 27.8089)
  arc A82 (41.3574, 28.0992) -> (44.4259, 27.8089) centre (43.0117, 29.2231) ccw
  arc A83 (41.3574, 28.0992) -> (28.0992, 41.3574) centre (0, 0) ccw
  arc A84 (27.8089, 44.4259) -> (28.0992, 41.3574) centre (29.2231, 43.0117) ccw
  line L52 (-38.3596, -35.7147) -> (-57.6913, -46.8758)
  arc A85 (-60.4233, -46.1437) -> (-57.6913, -46.8758) centre (-58.6913, -45.1437) ccw
  line L53 (-60.4233, -46.1437) -> (-70.1733, -29.2563)
  arc A86 (-69.4413, -26.5242) -> (-70.1733, -29.2563) centre (-68.4413, -28.2563) ccw
  line L54 (-69.4413, -26.5242) -> (-50.1096, -15.3631)
  arc A87 (-47.2208, -16.4376) -> (-50.1096, -15.3631) centre (-49.1096, -17.0951) ccw
  arc A88 (-47.2208, -16.4376) -> (-37.8458, -32.6756) centre (0, 0) ccw
  arc A89 (-38.3596, -35.7147) -> (-37.8458, -32.6756) centre (-39.3596, -33.9826) ccw
  arc A90 (-31.3739, -38.9317) -> (-28.1158, -41.3462) centre (0, 0) ccw
  arc A91 (-29.2404, -45) -> (-28.1158, -41.3462) centre (-29.2404, -43) ccw
  line L55 (-29.2404, -45) -> (-36.9782, -45)
  arc A92 (-37.9782, -41.2679) -> (-36.9782, -45) centre (-36.9782, -43) ccw
  line L56 (-37.9782, -41.2679) -> (-33.6289, -38.7569)
  arc A93 (-31.3739, -38.9317) -> (-33.6289, -38.7569) centre (-32.6289, -40.4889) ccw
  line L57 (80.1362, -12) -> (74.6733, -21.462)
  arc A94 (71.9413, -22.1941) -> (74.6733, -21.462) centre (72.9413, -20.462) ccw
  line L58 (71.9413, -22.1941) -> (55.6136, -12.7673)
  arc A95 (56.6098, -9.0353) -> (55.6136, -12.7673) centre (56.6136, -11.0353) ccw
  line L59 (56.6098, -9.0353) -> (75, -9)
  line L60 (75, -9) -> (78.4042, -9)
  arc A96 (80.1362, -12) -> (78.4042, -9) centre (78.4042, -11) ccw
  line L61 (-44.4259, 27.8089) -> (-60.2101, 43.5931)
  arc A97 (-60.2101, 46.4216) -> (-60.2101, 43.5931) centre (-58.7959, 45.0073) ccw
  line L62 (-60.2101, 46.4216) -> (-46.4216, 60.2101)
  arc A98 (-43.5931, 60.2101) -> (-46.4216, 60.2101) centre (-45.0073, 58.7959) ccw
  line L63 (-43.5931, 60.2101) -> (-27.8089, 44.4259)
  arc A99 (-28.0992, 41.3574) -> (-27.8089, 44.4259) centre (-29.2231, 43.0117) ccw
  arc A100 (-28.0992, 41.3574) -> (-41.3574, 28.0992) centre (0, 0) ccw
  arc A101 (-44.4259, 27.8089) -> (-41.3574, 28.0992) centre (-43.0117, 29.2231) ccw
  line L64 (50.1096, -15.3631) -> (69.4413, -26.5242)
  arc A102 (70.1733, -29.2563) -> (69.4413, -26.5242) centre (68.4413, -28.2563) ccw
  line L65 (70.1733, -29.2563) -> (60.4233, -46.1437)
  arc A103 (57.6913, -46.8758) -> (60.4233, -46.1437) centre (58.6913, -45.1437) ccw
  line L66 (57.6913, -46.8758) -> (38.3596, -35.7147)
  arc A104 (37.8458, -32.6756) -> (38.3596, -35.7147) centre (39.3596, -33.9826) ccw
  arc A105 (37.8458, -32.6756) -> (47.2208, -16.4376) centre (0, 0) ccw
  arc A106 (50.1096, -15.3631) -> (47.2208, -16.4376) centre (49.1096, -17.0951) ccw
  line L67 (-78.4041, -8.9935) -> (-56.6098, -9.0353)
  arc A107 (-55.6136, -12.7673) -> (-56.6098, -9.0353) centre (-56.6136, -11.0353) ccw
  line L68 (-55.6136, -12.7673) -> (-71.9413, -22.1941)
  arc A108 (-74.6733, -21.462) -> (-71.9413, -22.1941) centre (-72.9413, -20.462) ccw
  line L69 (-74.6733, -21.462) -> (-80.14, -11.9935)
  arc A109 (-78.4041, -8.9935) -> (-80.14, -11.9935) centre (-78.4079, -10.9935) ccw
  line L70 (33.6289, -38.7569) -> (37.9782, -41.268)
  arc A110 (36.9782, -45) -> (37.9782, -41.268) centre (36.9782, -43) ccw
  line L71 (36.9782, -45) -> (29.2404, -45)
  arc A111 (28.1158, -41.3462) -> (29.2404, -45) centre (29.2404, -43) ccw
  arc A112 (28.1158, -41.3462) -> (31.3739, -38.9317) centre (0, 0) ccw
  arc A113 (33.6289, -38.7569) -> (31.3739, -38.9317) centre (32.6289, -40.4889) ccw
  circle A114 centre (0, 0) radius 32
  circle A115 centre (-51.2451, -46.0409) radius 1.5
  circle A116 centre (51.2451, -46.0409) radius 1.5
  circle A117 centre (-65.4951, -21.3591) radius 1.5
  circle A118 centre (-57.7353, 37.5827) radius 1.5
  circle A119 centre (-37.5827, 57.7353) radius 1.5
  circle A120 centre (37.5827, 57.7353) radius 1.5
  circle A121 centre (57.7353, 37.5827) radius 1.5
  circle A122 centre (65.4951, -21.3591) radius 1.5
  arc A123 (46.6154, -4) -> (44.6318, -5.7447) centre (46.6154, -6) ccw
  arc A124 (34.9751, -28.3151) -> (44.6318, -5.7447) centre (0, 0) ccw
  arc A125 (32.0064, -28.4709) -> (34.9751, -28.3151) centre (33.4206, -27.0567) ccw
  line L72 (32.0064, -28.4709) -> (29.1607, -25.6252)
  arc A126 (29.007, -22.9694) -> (29.1607, -25.6252) centre (30.575, -24.211) ccw
  arc A127 (29.007, -22.9694) -> (29.007, 22.9694) centre (0, 0) ccw
  arc A128 (29.1607, 25.6252) -> (29.007, 22.9694) centre (30.575, 24.211) ccw
  line L73 (29.1607, 25.6252) -> (32.0064, 28.4709)
  arc A129 (34.9751, 28.3151) -> (32.0064, 28.4709) centre (33.4206, 27.0567) ccw
  arc A130 (44.6318, 5.7447) -> (34.9751, 28.3151) centre (0, 0) ccw
  arc A131 (44.6318, 5.7447) -> (46.6154, 4) centre (46.6154, 6) ccw
  line L74 (46.6154, 4) -> (96.9794, 4)
  arc A132 (98.979, 2.0412) -> (96.9794, 4) centre (96.9794, 2) ccw
  arc A133 (98.979, -2.0412) -> (98.979, 2.0412) centre (0, 0) ccw
  arc A134 (96.9794, -4) -> (98.979, -2.0412) centre (96.9794, -2) ccw
  line L75 (96.9794, -4) -> (46.6154, -4)
  arc A135 (-5.7447, 44.6318) -> (-4, 46.6154) centre (-6, 46.6154) ccw
  line L76 (-4, 46.6154) -> (-4, 96.9794)
  arc A136 (-2.0412, 98.979) -> (-4, 96.9794) centre (-2, 96.9794) ccw
  arc A137 (2.0412, 98.979) -> (-2.0412, 98.979) centre (0, 0) ccw
  arc A138 (4, 96.9794) -> (2.0412, 98.979) centre (2, 96.9794) ccw
  line L77 (4, 96.9794) -> (4, 46.6154)
  arc A139 (4, 46.6154) -> (5.7447, 44.6318) centre (6, 46.6154) ccw
  arc A140 (28.3151, 34.9751) -> (5.7447, 44.6318) centre (0, 0) ccw
  arc A141 (28.4709, 32.0064) -> (28.3151, 34.9751) centre (27.0567, 33.4206) ccw
  line L78 (28.4709, 32.0064) -> (25.6252, 29.1607)
  arc A142 (22.9694, 29.007) -> (25.6252, 29.1607) centre (24.211, 30.575) ccw
  arc A143 (22.9694, 29.007) -> (-22.9694, 29.007) centre (0, 0) ccw
  arc A144 (-25.6252, 29.1607) -> (-22.9694, 29.007) centre (-24.211, 30.575) ccw
  line L79 (-25.6252, 29.1607) -> (-28.4709, 32.0064)
  arc A145 (-28.3151, 34.9751) -> (-28.4709, 32.0064) centre (-27.0567, 33.4206) ccw
  arc A146 (-5.7447, 44.6318) -> (-28.3151, 34.9751) centre (0, 0) ccw
  arc A147 (31.3955, 80.893) -> (31.3955, 75.2362) centre (34.224, 78.0646) ccw
  line L80 (31.3955, 75.2362) -> (40.0576, 66.5741)
  arc A148 (40.0576, 63.7457) -> (40.0576, 66.5741) centre (38.6434, 65.1599) ccw
  line L81 (40.0576, 63.7457) -> (22.452, 46.1401)
  arc A149 (20.2286, 45.7253) -> (22.452, 46.1401) centre (21.0378, 47.5543) ccw
  arc A150 (20.2286, 45.7253) -> (10.5769, 48.8685) centre (0, 0) ccw
  arc A151 (9, 50.8232) -> (10.5769, 48.8685) centre (11, 50.8232) ccw
  line L82 (9, 50.8232) -> (9, 96.3743)
  arc A152 (11.2268, 98.3614) -> (9, 96.3743) centre (11, 96.3743) ccw
  arc A153 (38.0084, 91.4132) -> (11.2268, 98.3614) centre (0, 0) ccw
  arc A154 (38.6547, 88.1522) -> (38.0084, 91.4132) centre (37.2405, 89.5664) ccw
  line L83 (38.6547, 88.1522) -> (31.3955, 80.893)
  arc A155 (-31.3955, 75.2362) -> (-31.3955, 80.893) centre (-34.224, 78.0646) ccw
  line L84 (-31.3955, 80.893) -> (-38.6547, 88.1522)
  arc A156 (-38.0084, 91.4132) -> (-38.6547, 88.1522) centre (-37.2405, 89.5664) ccw
  arc A157 (-11.2268, 98.3614) -> (-38.0084, 91.4132) centre (0, 0) ccw
  arc A158 (-9, 96.3743) -> (-11.2268, 98.3614) centre (-11, 96.3743) ccw
  line L85 (-9, 96.3743) -> (-9, 50.8232)
  arc A159 (-10.5769, 48.8685) -> (-9, 50.8232) centre (-11, 50.8232) ccw
  arc A160 (-10.5769, 48.8685) -> (-20.2286, 45.7253) centre (0, 0) ccw
  arc A161 (-22.452, 46.1401) -> (-20.2286, 45.7253) centre (-21.0378, 47.5543) ccw
  line L86 (-22.452, 46.1401) -> (-40.0576, 63.7457)
  arc A162 (-40.0576, 66.5741) -> (-40.0576, 63.7457) centre (-38.6434, 65.1599) ccw
  line L87 (-40.0576, 66.5741) -> (-31.3955, 75.2362)
  arc A163 (-80.893, 31.3955) -> (-75.2362, 31.3955) centre (-78.0646, 34.224) ccw
  line L88 (-75.2362, 31.3955) -> (-66.5741, 40.0576)
  arc A164 (-63.7457, 40.0576) -> (-66.5741, 40.0576) centre (-65.1599, 38.6434) ccw
  line L89 (-63.7457, 40.0576) -> (-46.1401, 22.452)
  arc A165 (-45.7253, 20.2286) -> (-46.1401, 22.452) centre (-47.5543, 21.0378) ccw
  arc A166 (-45.7253, 20.2286) -> (-48.8685, 10.5769) centre (0, 0) ccw
  arc A167 (-50.8232, 9) -> (-48.8685, 10.5769) centre (-50.8232, 11) ccw
  line L90 (-50.8232, 9) -> (-96.3743, 9)
  arc A168 (-98.3614, 11.2268) -> (-96.3743, 9) centre (-96.3743, 11) ccw
  arc A169 (-91.4132, 38.0084) -> (-98.3614, 11.2268) centre (0, 0) ccw
  arc A170 (-88.1522, 38.6547) -> (-91.4132, 38.0084) centre (-89.5664, 37.2405) ccw
  line L91 (-88.1522, 38.6547) -> (-80.893, 31.3955)
  line L92 (40, -50) -> (-40, -50)
  line L93 (1, 17) -> (0.004, 17)
  line L94 (1, 16) -> (0.004, 16)
  line L95 (0.004, 16) -> (-23, 16)
  line L96 (-23, 16) -> (-23, -50)
  line L97 (0.004, 16) -> (23.004, 16)
  line L98 (23.004, 16) -> (23.004, -50)
  line L99 (40, -50) -> (23.004, -40.172)
  line L100 (-40, -50) -> (-23, -40.172)
  dimension "d202" = 80
  dimension "d203" = 23
  constraint parallel L20 L92
  constraint perpendicular L19 L93
  constraint parallel L93 L94
  constraint parallel L94 L95
  constraint coincident L24 L96.end
  constraint perpendicular L24 L96
  constraint perpendicular L96 L97
  constraint coincident L20 L98.end
  constraint perpendicular L20 L98
  constraint coincident L98 L99.end
  constraint coincident L96 L100.end
  measures "d202" distance of L92.start L92.end
  measures "d203" distance of L94.end L97.end
extrude "押し出し30" add sketch "スケッチ31" along normal blind 1.6 contours A27 A28 L24 A41 L25 L26 L92 L96 | A27 A28 A30 A31 A32 A34 A35 L19 A36 A41 L25 L26 L92 L96 L98 | A30 A31 A32 A114 L96 L98 | L24 A91 L55 L92 L96 L100 | A114 L94 L95 L96 L97 L98 | A91 L55 L100 | A34 A35 L19 A36 L20 L92 L98 | L20 L71 A111 L92 L98 L99 | L71 A111 L99 picked at (-15.332, 3.2505) bodies 1